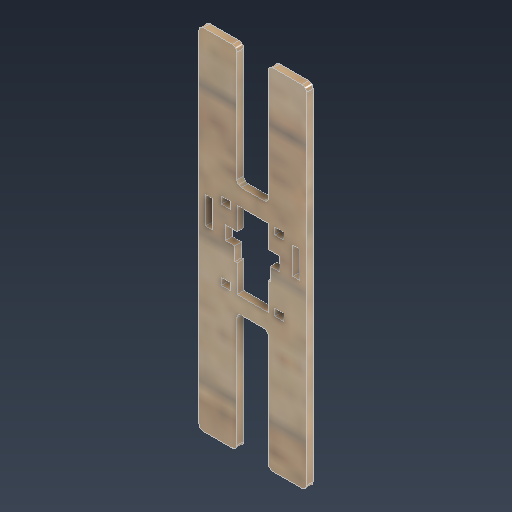
# Autodesk Inventor part: main_frame
Saved by Autodesk Inventor 2025.3 (Build 293356000, 356)
## iProperties
Created: 2025-09-03
Part Number: main_frame
Material: 木材 (楓木)
Document SubType Name: Modeling
Designer: 陳泓任
Density: 0.67 g/cm^3
Appearance: 天然楓木 - 深色亮面處理
Author: 陳泓任
Autodesk Inventor part; units mm, degrees
ref_plane "YZ Plane" through (0, 0, 0) normal (1, 0, 0) x (0, 1, 0)
ref_plane "XZ Plane" through (0, 0, 0) normal (0, 1, 0) x (-1, 0, 0)
ref_plane "XY Plane" through (0, 0, 0) normal (0, 0, 1) x (1, 0, 0)
sketch "草圖1" plane through (0, 0, 0) normal (0, 0, 1) x (1, 0, 0)
  line L0 (-23.85, -77.5) -> (23.85, 77.5) construction
  line L1 (23.85, -77.5) -> (-23.85, 77.5) construction
  line L2 (0, 127.6921) -> (0, -161.3915) construction
  line L3 (-23.85, 75.5) -> (-23.85, -75.5)
  line L4 (23.85, -75.5) -> (23.85, 75.5)
  line L5 (-5, 24.5) -> (5, 24.5)
  line L6 (7, 26.5) -> (7, 75.5)
  line L7 (-7, 75.5) -> (-7, 26.5)
  line L8 (-7, 24.5) -> (7, 77.5) construction
  line L9 (7, 24.5) -> (-7, 77.5) construction
  line L10 (21.85, 77.5) -> (9, 77.5)
  line L11 (-9, 77.5) -> (-21.85, 77.5)
  arc A0 (-7, 75.5) -> (-9, 77.5) centre (-9, 75.5) ccw
  arc A1 (9, 77.5) -> (7, 75.5) centre (9, 75.5) ccw
  arc A2 (-7, 26.5) -> (-5, 24.5) centre (-5, 26.5) ccw
  arc A3 (5, 24.5) -> (7, 26.5) centre (5, 26.5) ccw
  arc A4 (-21.85, 77.5) -> (-23.85, 75.5) centre (-21.85, 75.5) ccw
  arc A5 (23.85, 75.5) -> (21.85, 77.5) centre (21.85, 75.5) ccw
  line L12 (-82.8249, 0) -> (86.4934, 0) construction
  line L13 (-5, -24.5) -> (5, -24.5)
  line L14 (7, -26.5) -> (7, -75.5)
  line L15 (-7, -75.5) -> (-7, -26.5)
  line L16 (-7, -24.5) -> (7, -77.5) construction
  line L17 (7, -24.5) -> (-7, -77.5) construction
  line L18 (21.85, -77.5) -> (9, -77.5)
  line L19 (-9, -77.5) -> (-21.85, -77.5)
  arc A6 (-9, -77.5) -> (-7, -75.5) centre (-9, -75.5) ccw
  arc A7 (7, -75.5) -> (9, -77.5) centre (9, -75.5) ccw
  arc A8 (-5, -24.5) -> (-7, -26.5) centre (-5, -26.5) ccw
  arc A9 (7, -26.5) -> (5, -24.5) centre (5, -26.5) ccw
  arc A10 (-23.85, -75.5) -> (-21.85, -77.5) centre (-21.85, -75.5) ccw
  arc A11 (21.85, -77.5) -> (23.85, -75.5) centre (21.85, -75.5) ccw
  line L20 (-21.85, -77.5) -> (-9, -77.5)
  line L21 (9, -77.5) -> (21.85, -77.5)
  line L22 (-6.85, -17.45) -> (6.85, -17.45)
  line L23 (6.85, 16.75) -> (-6.85, 16.75)
  line L24 (12.065, 0.7) -> (12.065, 6.7)
  line L25 (-12.065, 6.7) -> (-12.065, 0.7)
  line L26 (-12.065, 0.7) -> (12.065, 6.7) construction
  line L27 (12.065, 0.7) -> (-12.065, 6.7) construction
  line L28 (-6.85, 16.75) -> (-6.85, 6.7)
  line L29 (6.85, 6.7) -> (6.85, 16.75)
  line L30 (12.065, 6.7) -> (6.85, 6.7)
  line L31 (7.85, 0.7) -> (12.065, 0.7)
  line L32 (-12.065, 0.7) -> (-7.85, 0.7)
  line L33 (-6.85, 6.7) -> (-12.065, 6.7)
  line L34 (-7.85, 0.7) -> (-7.85, -5.3)
  line L35 (-7.85, -5.3) -> (-6.85, -5.3)
  line L36 (-6.85, -5.3) -> (-6.85, -17.45)
  line L37 (7.85, 0.7) -> (7.85, -5.3)
  line L38 (7.85, -5.3) -> (6.85, -5.3)
  line L39 (6.85, -17.45) -> (6.85, -5.3)
  point P0 (0, 0)
  point P1 (0, 51)
  point P2 (0, -51)
  point P3 (0, 3.7)
  point P4 (12.065, 3.7)
  point P5 (-23.85, -75.5)
  dimension "d0" = 47.7
  dimension "d22" = 14
  dimension "d24" = 2
  dimension "d25" = 2
  dimension "d26" = 34.2
  dimension "d27" = 13.7
  dimension "d28" = 6
  dimension "d30" = 24.13
  dimension "d31" = 10.05
  dimension "d54" = 53
  dimension "d97" = 6
  dimension "d98" = 1
  dimension "d101" = 0.7
  dimension "d103" = 155
  constraints: 80 end point, 27 symmetric about line, 26 point on line, 24 point on circle, 16 parallel, 12 centre point, 12 tangent, 9 perpendicular, 7 horizontal, 7 midpoint, 4 equal radius, 2 collinear, 1 vertical, 8 other
  measures "d0" distance of L0.end L1.end
  measures "d22" distance of L8.start L9.start
  measures "d24" radius of A0
  measures "d25" radius of A4
  measures "d26" distance of L22.end L23.start
  measures "d27" distance of L23.start L23.end
  measures "d28" distance of L24.start L24.end
  measures "d30" distance from line of point (12.065, 3.7) L25
  measures "d31" distance between parallel lines of L33 L23
  measures "d54" distance between parallel lines of L11 L5
  measures "d97" distance of L32.end L34.end
  measures "d98" distance of L34.end L35.end
  measures "d101" distance between parallel lines of L12 L32
  measures "d103" distance between parallel lines of L18 L10
extrude "擠出1" add sketch "草圖1" along normal blind 3
sketch "草圖3" plane through (0, 0, 3) normal (0, 0, 1) x (1, 0, 0)
  line L0 (-88.1264, 0) -> (75.7938, 0)
  line L1 (0, 123.8394) -> (0, -129.4918)
  point P0 (0, 0)
  constraints: 4 end point, 2 point on line, 1 horizontal, 1 perpendicular
sketch "草圖5" plane through (0, 0, 3) normal (0, 0, 1) x (1, 0, 0)
  line L0 (-9.85, -17.45) -> (-13.85, -17.45)
  line L1 (-13.85, -17.45) -> (-13.85, -14.45)
  line L2 (-13.85, -14.45) -> (-9.85, -14.45)
  line L3 (-9.85, -14.45) -> (-9.85, -17.45)
  line L4 (6.85, -17.45) -> (-6.85, -17.45) projected
  line L5 (-9.85, 13.75) -> (-13.85, 13.75)
  line L6 (-13.85, 13.75) -> (-13.85, 16.75)
  line L7 (-13.85, 16.75) -> (-9.85, 16.75)
  line L8 (-9.85, 16.75) -> (-9.85, 13.75)
  line L9 (-6.85, 16.75) -> (6.85, 16.75) projected
  line L10 (0, 31.1544) -> (0, -25.4134)
  line L11 (9.85, -17.45) -> (13.85, -17.45)
  line L12 (13.85, -17.45) -> (13.85, -14.45)
  line L13 (13.85, -14.45) -> (9.85, -14.45)
  line L14 (9.85, -14.45) -> (9.85, -17.45)
  line L15 (13.85, 16.75) -> (9.85, 16.75)
  line L16 (13.85, 13.75) -> (13.85, 16.75)
  line L17 (9.85, 13.75) -> (13.85, 13.75)
  line L18 (9.85, 16.75) -> (9.85, 13.75)
  line L19 (-17.85, 1.825) -> (-20.85, 1.825)
  line L20 (-20.85, 1.825) -> (-20.85, 13.825)
  line L21 (-20.85, 13.825) -> (-17.85, 13.825)
  line L22 (-17.85, 13.825) -> (-17.85, 1.825)
  line L23 (17.85, 1.825) -> (20.85, 1.825)
  line L24 (20.85, 1.825) -> (20.85, 13.825)
  line L25 (20.85, 13.825) -> (17.85, 13.825)
  line L26 (17.85, 13.825) -> (17.85, 1.825)
  line L27 (-6.85, -17.45) -> (-6.85, 16.75) construction
  point P0 (0, 0)
  dimension "d60" = 4
  dimension "d62" = 3
  dimension "d64" = 3
  dimension "d66" = 3
  dimension "d67" = 12
  dimension "d96" = 3
  dimension "d100" = 11
  dimension "d102" = 0.075
  constraints: 52 end point, 12 symmetric about line, 6 parallel, 4 collinear, 3 horizontal, 3 perpendicular, 1 point on line, 1 vertical
  measures "d60" distance of L0.start L0.end
  measures "d62" distance of L0.end L1.end
  measures "d64" distance of L6.start L7.start
  measures "d66" distance of L20.end L21.end
  measures "d67" distance of L21.end L19.start
  measures "d96" distance between parallel lines of L27 L3
  measures "d100" distance between parallel lines of L27 L22
  measures "d102" distance between parallel lines of L5 L21
extrude "擠出4" cut sketch "草圖5" against normal up to next
